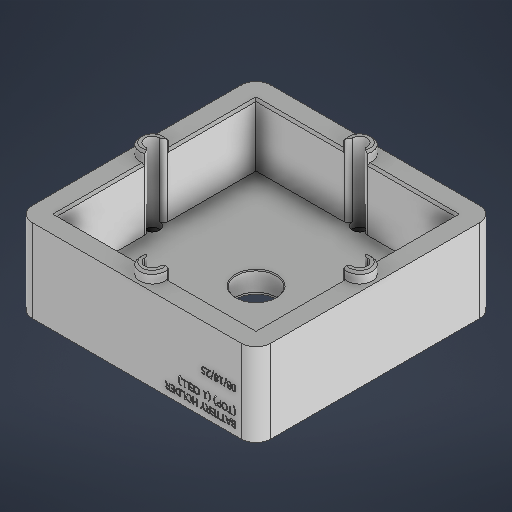
# Autodesk Inventor part: Battery Holder (Top)
Saved by Autodesk Inventor 2025 (Build 290162000, 162)
## iProperties
Created: 2025-08-08
Part Number: Battery Holder (Top)
Material: Generic
Document SubType Name: Modeling
Designer: mayhe
Density: 1 g/cm^3
Appearance: Default
Author: mayhe
Autodesk Inventor part; units mm, degrees
ref_plane "YZ Plane" through (0, 0, 0) normal (1, 0, 0) x (0, 1, 0)
ref_plane "XZ Plane" through (0, 0, 0) normal (0, 1, 0) x (-1, 0, 0)
ref_plane "XY Plane" through (0, 0, 0) normal (0, 0, 1) x (1, 0, 0)
sketch "Sketch1" plane through (0, 0, 0) normal (0, 1, 0) x (-1, 0, 0)
  line L0 (57.5, 57.5) -> (-57.5, 57.5)
  line L1 (-57.5, 57.5) -> (-57.5, -57.5)
  line L2 (-57.5, -57.5) -> (57.5, -57.5)
  line L3 (57.5, -57.5) -> (57.5, 57.5)
  line L4 (57.5, 57.5) -> (-57.5, -57.5) construction
  line L5 (-57.5, 57.5) -> (57.5, -57.5) construction
  point P0 (0, 0)
  dimension "d0" = 115
  dimension "d1" = 115
  constraints: 12 end point, 2 midpoint, 2 parallel, 1 horizontal, 1 perpendicular
  measures "d0" distance of L2.end L1.end
  measures "d1" distance of L1.end L0.end
extrude "Extrusion1" add sketch "Sketch1" along normal blind 10
sketch "Sketch4" plane through (0, 10, 0) normal (0, 1, 0) x (1, 0, 0)
  line L0 (-48, -48) -> (48, -48)
  line L1 (48, -48) -> (48, 48)
  line L2 (48, 48) -> (-48, 48)
  line L3 (-48, 48) -> (-48, -48)
  line L4 (-57.5, 57.5) -> (-57.5, -57.5) projected
  line L5 (-57.5, 0) -> (-48, 0)
  line L6 (-57.5, -57.5) -> (57.5, -57.5) projected
  line L7 (-57.5, 57.5) -> (57.5, 57.5)
  line L8 (57.5, 57.5) -> (57.5, -57.5)
  line L9 (57.5, -57.5) -> (-57.5, -57.5)
  line L10 (-57.5, -57.5) -> (-57.5, 57.5)
  circle A0 centre (0, 0) radius 9.5
  point P0 (47.3285, -94.6135)
  point P1 (-53.5957, 219.1108)
  point P2 (48, 0)
  point P3 (0, -48)
  point P4 (0, -57.5)
  dimension "d48" = 96
  dimension "d49" = 96
  dimension "d217" = 19
  constraints: 18 end point, 6 midpoint, 4 parallel, 2 horizontal, 2 perpendicular, 1 centre point, 1 horizontal alignment, 1 vertical alignment
  measures "d48" distance of L2.end L1.end
  measures "d49" distance of L1.end L0.end
  measures "d217" diameter of A0
extrude "Extrusion3" add sketch "Sketch4" along normal blind 30 contours L7 L8 L6 L4
hole "Hole4" at (0, 10, 0) direction (0, -1, 0) diameter 18.6 end through all countersink diameter 19 countersink angle 2.5
sketch "Sketch6" plane through (0, 0, 0) normal (0, -1, 0) x (1, 0, 0)
  line L0 (50, 50) -> (-50, 50)
  line L1 (-50, 50) -> (-50, -50)
  line L2 (-50, -50) -> (50, -50)
  line L3 (50, -50) -> (50, 50)
  line L4 (50, 50) -> (-50, -50) construction
  line L5 (-50, 50) -> (50, -50) construction
  circle A0 centre (-50, -50) radius 3
  circle A1 centre (0, -50) radius 3
  circle A2 centre (50, -50) radius 3
  circle A3 centre (-50, 0) radius 3
  circle A4 centre (0, 0) radius 3
  circle A5 centre (50, 0) radius 3
  circle A6 centre (-50, 50) radius 3
  circle A7 centre (0, 50) radius 3
  circle A8 centre (50, 50) radius 3
  dimension "d183" = 100
  dimension "d184" = 100
  dimension "d185" = 6
  dimension "d188" = 50
  dimension "d191" = 50
  constraints: 12 end point, 9 centre point, 2 horizontal, 2 midpoint, 2 parallel, 1 coincident, 1 perpendicular, 1 vertical, 16 other
  measures "d183" distance of L2.end L1.end
  measures "d184" distance of L1.end L0.end
  measures "d185" diameter of A0
  measures "d188" distance of A0.centre A1.centre
  measures "d191" distance of A0.centre A3.centre
hole "Hole5" at (-50, 0, 0) at (0, 0, -50) at (50, 0, 0) at (0, 0, 50) direction (0, 1, 0) diameter 7.125 end through all counterbore diameter 13 counterbore depth 7
sketch "Sketch7" plane through (0, 40, 0) normal (0, 1, 0) x (1, 0, 0)
  arc A0 (-48, 2.9481) -> (-48, -2.9481) centre (-50, 0) ccw projected
  arc A1 (-48, 5.6569) -> (-48, -5.6569) centre (-50, 0) ccw
  circle A2 centre (50, 0) radius 6.5 projected
  arc A3 (48, -5.6569) -> (48, 5.6569) centre (50, 0) ccw
  circle A4 centre (0, 50) radius 3.5625 projected
  arc A5 (5.6569, 48) -> (-5.6569, 48) centre (0, 50) ccw
  arc A6 (-2.9481, -48) -> (2.9481, -48) centre (0, -50) ccw projected
  arc A7 (-5.6569, -48) -> (5.6569, -48) centre (0, -50) ccw
  line L0 (-2.9481, 48) -> (-48, 48) projected
  line L1 (48, -48) -> (2.9481, -48) projected
  line L2 (-48, 48) -> (48, 48)
  line L3 (48, 48) -> (48, -48)
  line L4 (48, -48) -> (-48, -48)
  line L5 (-48, -48) -> (-48, 48)
  arc A8 (-48, 2.9481) -> (-48, -2.9481) centre (-50, 0) ccw
  arc A9 (-2.9481, -48) -> (2.9481, -48) centre (0, -50) ccw
  arc A10 (48, -2.9481) -> (48, 2.9481) centre (50, 0) ccw
  arc A11 (2.9481, 48) -> (-2.9481, 48) centre (0, 50) ccw
  point P0 (0, 0)
  point P1 (-48, 2.9481)
  point P2 (-48, -2.9481)
  point P3 (-2.9481, -48)
  point P4 (5.6569, -48)
  point P5 (-5.6569, 48)
  dimension "d201" = 12
  dimension "d202" = 12
  dimension "d203" = 12
  dimension "d204" = 12
  constraints: 16 point on circle, 16 point on line, 8 centre point, 8 coincident, 8 end point, 2 concentric, 2 parallel, 1 horizontal, 1 perpendicular, 2 other
  measures "d201" diameter of A1
  measures "d202" diameter of A3
  measures "d203" diameter of A5
  measures "d204" diameter of A7
extrude "Extrusion4" add sketch "Sketch7" along normal blind 5 contours A0 L5 A1 | A5 L2 A4 L0 | L4 A6 L1 A7 | A3 L3 A10
fillet "Fillet1" radius 7.125 4 edges at (-57.5, 20, -57.5) (57.5, 20, -57.5) (57.5, 20, 57.5) (-57.5, 20, 57.5)
fillet "Fillet2" radius 2 16 edges at (2.9481, 25, -48) (-2.9481, 42.5, -48) (-2.9481, 25, -48) (2.9481, 42.5, -48) (48, 25, 2.9481) (48, 42.5, -2.9481) (48, 25, -2.9481) (48, 42.5, 2.9481) (2.9481, 42.5, 48) (2.9481, 25, 48) (-2.9481, 25, 48) (-2.9481, 42.5, 48) (-48, 25, -2.9481) (-48, 42.5, 2.9481) (-48, 25, 2.9481) (-48, 42.5, -2.9481)
chamfer "Chamfer1" distance 0.4 angle 45 1 edges at (0, 10, -9.5)
chamfer "Chamfer2" distance 1 angle 45 12 edges at (0, 45, -56) (-56, 45, 0) (0, 45, 56) (56, 45, 0) (-26.8284, 40, -48) (-48, 40, -26.8284) (48, 40, -26.8284) (26.8284, 40, -48) (48, 40, 26.8284) (26.8284, 40, 48) (-26.8284, 40, 48) (-48, 40, 26.8284)
sketch "Sketch8" plane through (-50.375, 0, 57.5) normal (0, 0, 1) x (1, 0, 0)
  line L0 (98.2962, 2.8919) -> (49.8661, 2.8919) construction
  line L1 (49.8661, 2.8919) -> (49.8661, 31.9849) construction
  line L2 (49.8661, 31.9849) -> (98.2962, 31.9849) construction
  line L3 (98.2962, 31.9849) -> (98.2962, 2.8919) construction
  spline S0 degree 2 poles (95.92, 5.068) (95.92, 5.2953) (96.0929, 5.6435) (96.2362, 5.7572) knots 0 0 0 1 2 2 2
  spline S1 degree 2 poles (96.2362, 5.7572) (96.4091, 5.8905) (96.8018, 6.0042) (97.113, 6.0042) knots 0 0 0 1 2 2 2
  line L4 (97.113, 6.0042) -> (97.9874, 6.0042)
  line L5 (97.9874, 6.0042) -> (97.9874, 2.9562)
  line L6 (97.9874, 2.9562) -> (97.1797, 2.9562)
  spline S2 degree 2 poles (97.1797, 2.9562) (96.8537, 2.9562) (96.5276, 2.9981) (96.3794, 3.0797) knots 0 0 0 1 2 2 2
  spline S3 degree 2 poles (96.3794, 3.0797) (96.2139, 3.1661) (96.0633, 3.4502) (96.0633, 3.6428) knots 0 0 0 1 2 2 2
  spline S4 degree 2 poles (96.0633, 3.6428) (96.0633, 3.8577) (96.2905, 4.1986) (96.4906, 4.2949) knots 0 0 0 1 2 2 2
  line L7 (96.4906, 4.2949) -> (96.4906, 4.3097)
  spline S5 degree 2 poles (96.4906, 4.3097) (96.2189, 4.3838) (95.92, 4.7766) (95.92, 5.068) knots 0 0 0 1 2 2 2
  spline S6 degree 2 poles (96.3424, 5.0853) (96.3424, 4.9124) (96.4412, 4.6901) (96.5894, 4.6111) knots 0 0 0 1 2 2 2
  spline S7 degree 2 poles (96.5894, 4.6111) (96.6857, 4.5617) (96.913, 4.532) (97.1229, 4.532) knots 0 0 0 1 2 2 2
  line L8 (97.1229, 4.532) -> (97.5823, 4.532)
  line L9 (97.5823, 4.532) -> (97.5823, 5.6584)
  line L10 (97.5823, 5.6584) -> (97.2538, 5.6584)
  spline S8 degree 2 poles (97.2538, 5.6584) (96.9871, 5.6584) (96.6808, 5.609) (96.5622, 5.5299) knots 0 0 0 1 2 2 2
  spline S9 degree 2 poles (96.5622, 5.5299) (96.4486, 5.4484) (96.3424, 5.2459) (96.3424, 5.0853) knots 0 0 0 1 2 2 2
  spline S10 degree 2 poles (96.4856, 3.6996) (96.4856, 3.591) (96.5598, 3.4279) (96.6413, 3.381) knots 0 0 0 1 2 2 2
  spline S11 degree 2 poles (96.6413, 3.381) (96.7401, 3.3267) (96.9797, 3.302) (97.1945, 3.302) knots 0 0 0 1 2 2 2
  line L11 (97.1945, 3.302) -> (97.5823, 3.302)
  line L12 (97.5823, 3.302) -> (97.5823, 4.1936)
  line L13 (97.5823, 4.1936) -> (97.1229, 4.1936)
  spline S12 degree 2 poles (97.1229, 4.1936) (96.9327, 4.1936) (96.7524, 4.1541) (96.6561, 4.0924) knots 0 0 0 1 2 2 2
  spline S13 degree 2 poles (96.6561, 4.0924) (96.5622, 4.0331) (96.4856, 3.8429) (96.4856, 3.6996) knots 0 0 0 1 2 2 2
  line L14 (95.8459, 6.0042) -> (94.8184, 2.9562)
  line L15 (94.8184, 2.9562) -> (94.3194, 2.9562)
  line L16 (94.3194, 2.9562) -> (93.2919, 6.0042)
  line L17 (93.2919, 6.0042) -> (93.7192, 6.0042)
  line L18 (93.7192, 6.0042) -> (93.9959, 5.152)
  line L19 (93.9959, 5.152) -> (95.1593, 5.152)
  line L20 (95.1593, 5.152) -> (95.4359, 6.0042)
  line L21 (95.4359, 6.0042) -> (95.8459, 6.0042)
  line L22 (94.107, 4.8062) -> (94.5788, 3.3711)
  line L23 (94.5788, 3.3711) -> (95.0481, 4.8062)
  line L24 (95.0481, 4.8062) -> (94.107, 4.8062)
  line L25 (92.2916, 6.0042) -> (92.2916, 3.3168)
  line L26 (92.2916, 3.3168) -> (93.3141, 3.3168)
  line L27 (93.3141, 3.3168) -> (93.3141, 2.9562)
  line L28 (93.3141, 2.9562) -> (90.8639, 2.9562)
  line L29 (90.8639, 2.9562) -> (90.8639, 3.3168)
  line L30 (90.8639, 3.3168) -> (91.8865, 3.3168)
  line L31 (91.8865, 3.3168) -> (91.8865, 6.0042)
  line L32 (91.8865, 6.0042) -> (92.2916, 6.0042)
  line L33 (89.8438, 6.0042) -> (89.8438, 3.3168)
  line L34 (89.8438, 3.3168) -> (90.8664, 3.3168)
  line L35 (90.8664, 3.3168) -> (90.8664, 2.9562)
  line L36 (90.8664, 2.9562) -> (88.4161, 2.9562)
  line L37 (88.4161, 2.9562) -> (88.4161, 3.3168)
  line L38 (88.4161, 3.3168) -> (89.4387, 3.3168)
  line L39 (89.4387, 3.3168) -> (89.4387, 6.0042)
  line L40 (89.4387, 6.0042) -> (89.8438, 6.0042)
  line L41 (88.1074, 6.0042) -> (88.1074, 2.9562)
  line L42 (88.1074, 2.9562) -> (86.2005, 2.9562)
  line L43 (86.2005, 2.9562) -> (86.2005, 3.3168)
  line L44 (86.2005, 3.3168) -> (87.7023, 3.3168)
  line L45 (87.7023, 3.3168) -> (87.7023, 4.1516)
  line L46 (87.7023, 4.1516) -> (86.3018, 4.1516)
  line L47 (86.3018, 4.1516) -> (86.3018, 4.5123)
  line L48 (86.3018, 4.5123) -> (87.7023, 4.5123)
  line L49 (87.7023, 4.5123) -> (87.7023, 5.6435)
  line L50 (87.7023, 5.6435) -> (86.2005, 5.6435)
  line L51 (86.2005, 5.6435) -> (86.2005, 6.0042)
  line L52 (86.2005, 6.0042) -> (88.1074, 6.0042)
  line L53 (83.397, 6.0042) -> (83.9231, 6.0042)
  line L54 (83.9231, 6.0042) -> (84.8865, 4.7914)
  line L55 (84.8865, 4.7914) -> (85.3508, 4.7914)
  line L56 (85.3508, 4.7914) -> (85.3508, 6.0042)
  line L57 (85.3508, 6.0042) -> (85.7559, 6.0042)
  line L58 (85.7559, 6.0042) -> (85.7559, 2.9562)
  line L59 (85.7559, 2.9562) -> (84.9704, 2.9562)
  spline S14 degree 2 poles (84.9704, 2.9562) (84.7086, 2.9562) (84.3554, 3.013) (84.1948, 3.1167) knots 0 0 0 1 2 2 2
  spline S15 degree 2 poles (84.1948, 3.1167) (84.0343, 3.2204) (83.849, 3.544) (83.849, 3.7836) knots 0 0 0 1 2 2 2
  spline S16 degree 2 poles (83.849, 3.7836) (83.849, 4.1171) (84.1899, 4.5691) (84.4814, 4.6778) knots 0 0 0 1 2 2 2
  line L60 (84.4814, 4.6778) -> (83.397, 6.0042)
  spline S17 degree 2 poles (84.2714, 3.8157) (84.2714, 3.6823) (84.3653, 3.4773) (84.4641, 3.4106) knots 0 0 0 1 2 2 2
  spline S18 degree 2 poles (84.4641, 3.4106) (84.5505, 3.3538) (84.7802, 3.3069) (84.9482, 3.3069) knots 0 0 0 1 2 2 2
  line L61 (84.9482, 3.3069) -> (85.3508, 3.3069)
  line L62 (85.3508, 3.3069) -> (85.3508, 4.453)
  line L63 (85.3508, 4.453) -> (84.9951, 4.453)
  spline S19 degree 2 poles (84.9951, 4.453) (84.8198, 4.453) (84.5407, 4.3912) (84.4443, 4.2949) knots 0 0 0 1 2 2 2
  spline S20 degree 2 poles (84.4443, 4.2949) (84.3554, 4.2109) (84.2714, 3.9738) (84.2714, 3.8157) knots 0 0 0 1 2 2 2
  line L64 (81.0209, 2.9562) -> (82.0509, 4.6555)
  line L65 (82.0509, 4.6555) -> (82.0509, 6.0042)
  line L66 (82.0509, 6.0042) -> (82.456, 6.0042)
  line L67 (82.456, 6.0042) -> (82.456, 4.6975)
  line L68 (82.456, 4.6975) -> (83.486, 2.9562)
  line L69 (83.486, 2.9562) -> (83.0364, 2.9562)
  line L70 (83.0364, 2.9562) -> (82.2485, 4.2974)
  line L71 (82.2485, 4.2974) -> (81.4507, 2.9562)
  line L72 (81.4507, 2.9562) -> (81.0209, 2.9562)
  line L73 (77.2171, 6.0042) -> (77.6221, 6.0042)
  line L74 (77.6221, 6.0042) -> (77.6221, 4.5123)
  line L75 (77.6221, 4.5123) -> (79.0251, 4.5123)
  line L76 (79.0251, 4.5123) -> (79.0251, 6.0042)
  line L77 (79.0251, 6.0042) -> (79.4302, 6.0042)
  line L78 (79.4302, 6.0042) -> (79.4302, 2.9562)
  line L79 (79.4302, 2.9562) -> (79.0251, 2.9562)
  line L80 (79.0251, 2.9562) -> (79.0251, 4.1516)
  line L81 (79.0251, 4.1516) -> (77.6221, 4.1516)
  line L82 (77.6221, 4.1516) -> (77.6221, 2.9562)
  line L83 (77.6221, 2.9562) -> (77.2171, 2.9562)
  line L84 (77.2171, 2.9562) -> (77.2171, 6.0042)
  spline S21 degree 2 poles (74.4432, 3.3044) (74.2703, 3.507) (74.0777, 4.0998) (74.0777, 4.4802) knots 0 0 0 1 2 2 2
  spline S22 degree 2 poles (74.0777, 4.4802) (74.0777, 4.8507) (74.2654, 5.4509) (74.4432, 5.6534) knots 0 0 0 1 2 2 2
  spline S23 degree 2 poles (74.4432, 5.6534) (74.6309, 5.8658) (75.1274, 6.0684) (75.4263, 6.0684) knots 0 0 0 1 2 2 2
  spline S24 degree 2 poles (75.4263, 6.0684) (75.735, 6.0684) (76.229, 5.8584) (76.4094, 5.6534) knots 0 0 0 1 2 2 2
  spline S25 degree 2 poles (76.4094, 5.6534) (76.5847, 5.4509) (76.7725, 4.8556) (76.7725, 4.4802) knots 0 0 0 1 2 2 2
  spline S26 degree 2 poles (76.7725, 4.4802) (76.7725, 4.0973) (76.5823, 3.5144) (76.4069, 3.3044) knots 0 0 0 1 2 2 2
  spline S27 degree 2 poles (76.4069, 3.3044) (76.229, 3.1019) (75.7326, 2.8919) (75.4263, 2.8919) knots 0 0 0 1 2 2 2
  spline S28 degree 2 poles (75.4263, 2.8919) (75.1151, 2.8919) (74.6161, 3.1093) (74.4432, 3.3044) knots 0 0 0 1 2 2 2
  spline S29 degree 2 poles (74.5, 4.4802) (74.5, 4.1788) (74.6309, 3.712) (74.7495, 3.5588) knots 0 0 0 1 2 2 2
  spline S30 degree 2 poles (74.7495, 3.5588) (74.8705, 3.4008) (75.2114, 3.2427) (75.4238, 3.2427) knots 0 0 0 1 2 2 2
  spline S31 degree 2 poles (75.4238, 3.2427) (75.6437, 3.2427) (75.9746, 3.3958) (76.1006, 3.5588) knots 0 0 0 1 2 2 2
  spline S32 degree 2 poles (76.1006, 3.5588) (76.2216, 3.7145) (76.3501, 4.1838) (76.3501, 4.4802) knots 0 0 0 1 2 2 2
  spline S33 degree 2 poles (76.3501, 4.4802) (76.3501, 5.0804) (75.8462, 5.7176) (75.4238, 5.7176) knots 0 0 0 1 2 2 2
  spline S34 degree 2 poles (75.4238, 5.7176) (75.0014, 5.7176) (74.5, 5.0804) (74.5, 4.4802) knots 0 0 0 1 2 2 2
  line L85 (71.867, 6.0042) -> (73.6331, 6.0042)
  line L86 (73.6331, 6.0042) -> (73.6331, 2.9562)
  line L87 (73.6331, 2.9562) -> (73.228, 2.9562)
  line L88 (73.228, 2.9562) -> (73.228, 5.6435)
  line L89 (73.228, 5.6435) -> (71.867, 5.6435)
  line L90 (71.867, 5.6435) -> (71.867, 6.0042)
  spline S35 degree 2 poles (69.145, 4.4826) (69.145, 4.9001) (69.4834, 5.5719) (69.7675, 5.7596) knots 0 0 0 1 2 2 2
  spline S36 degree 2 poles (69.7675, 5.7596) (69.9997, 5.9054) (70.4764, 6.0042) (70.8469, 6.0042) knots 0 0 0 1 2 2 2
  line L91 (70.8469, 6.0042) -> (71.5484, 6.0042)
  line L92 (71.5484, 6.0042) -> (71.5484, 2.9562)
  line L93 (71.5484, 2.9562) -> (70.8543, 2.9562)
  spline S37 degree 2 poles (70.8543, 2.9562) (70.4245, 2.9562) (69.9354, 3.0846) (69.7625, 3.1982) knots 0 0 0 1 2 2 2
  spline S38 degree 2 poles (69.7625, 3.1982) (69.4686, 3.3933) (69.145, 4.038) (69.145, 4.4826) knots 0 0 0 1 2 2 2
  spline S39 degree 2 poles (69.5674, 4.4777) (69.5674, 4.1269) (69.7996, 3.6305) (70.0293, 3.4897) knots 0 0 0 1 2 2 2
  spline S40 degree 2 poles (70.0293, 3.4897) (70.1923, 3.3933) (70.5604, 3.3069) (70.8345, 3.3069) knots 0 0 0 1 2 2 2
  line L94 (70.8345, 3.3069) -> (71.1433, 3.3069)
  line L95 (71.1433, 3.3069) -> (71.1433, 5.6534)
  line L96 (71.1433, 5.6534) -> (70.8345, 5.6534)
  spline S41 degree 2 poles (70.8345, 5.6534) (70.5653, 5.6534) (70.1577, 5.567) (69.9923, 5.4509) knots 0 0 0 1 2 2 2
  spline S42 degree 2 poles (69.9923, 5.4509) (69.7798, 5.3076) (69.5674, 4.8334) (69.5674, 4.4777) knots 0 0 0 1 2 2 2
  line L97 (68.7054, 6.0042) -> (68.7054, 2.9562)
  line L98 (68.7054, 2.9562) -> (66.7985, 2.9562)
  line L99 (66.7985, 2.9562) -> (66.7985, 3.3168)
  line L100 (66.7985, 3.3168) -> (68.3003, 3.3168)
  line L101 (68.3003, 3.3168) -> (68.3003, 4.1516)
  line L102 (68.3003, 4.1516) -> (66.8998, 4.1516)
  line L103 (66.8998, 4.1516) -> (66.8998, 4.5123)
  line L104 (66.8998, 4.5123) -> (68.3003, 4.5123)
  line L105 (68.3003, 4.5123) -> (68.3003, 5.6435)
  line L106 (68.3003, 5.6435) -> (66.7985, 5.6435)
  line L107 (66.7985, 5.6435) -> (66.7985, 6.0042)
  line L108 (66.7985, 6.0042) -> (68.7054, 6.0042)
  line L109 (63.9951, 6.0042) -> (64.5212, 6.0042)
  line L110 (64.5212, 6.0042) -> (65.4845, 4.7914)
  line L111 (65.4845, 4.7914) -> (65.9488, 4.7914)
  line L112 (65.9488, 4.7914) -> (65.9488, 6.0042)
  line L113 (65.9488, 6.0042) -> (66.3539, 6.0042)
  line L114 (66.3539, 6.0042) -> (66.3539, 2.9562)
  line L115 (66.3539, 2.9562) -> (65.5685, 2.9562)
  spline S43 degree 2 poles (65.5685, 2.9562) (65.3066, 2.9562) (64.9534, 3.013) (64.7929, 3.1167) knots 0 0 0 1 2 2 2
  spline S44 degree 2 poles (64.7929, 3.1167) (64.6323, 3.2204) (64.4471, 3.544) (64.4471, 3.7836) knots 0 0 0 1 2 2 2
  spline S45 degree 2 poles (64.4471, 3.7836) (64.4471, 4.1171) (64.7879, 4.5691) (65.0794, 4.6778) knots 0 0 0 1 2 2 2
  line L116 (65.0794, 4.6778) -> (63.9951, 6.0042)
  spline S46 degree 2 poles (64.8694, 3.8157) (64.8694, 3.6823) (64.9633, 3.4773) (65.0621, 3.4106) knots 0 0 0 1 2 2 2
  spline S47 degree 2 poles (65.0621, 3.4106) (65.1486, 3.3538) (65.3783, 3.3069) (65.5462, 3.3069) knots 0 0 0 1 2 2 2
  line L117 (65.5462, 3.3069) -> (65.9488, 3.3069)
  line L118 (65.9488, 3.3069) -> (65.9488, 4.453)
  line L119 (65.9488, 4.453) -> (65.5932, 4.453)
  spline S48 degree 2 poles (65.5932, 4.453) (65.4178, 4.453) (65.1387, 4.3912) (65.0423, 4.2949) knots 0 0 0 1 2 2 2
  spline S49 degree 2 poles (65.0423, 4.2949) (64.9534, 4.2109) (64.8694, 3.9738) (64.8694, 3.8157) knots 0 0 0 1 2 2 2
  line L120 (96.8438, 11.8649) -> (97.3131, 11.8649)
  spline S50 degree 2 poles (97.3131, 11.8649) (97.6688, 11.4425) (98.0763, 10.4965) (98.0763, 9.8518) knots 0 0 0 1 2 2 2
  spline S51 degree 2 poles (98.0763, 9.8518) (98.0763, 9.222) (97.6737, 8.2611) (97.3131, 7.8388) knots 0 0 0 1 2 2 2
  line L121 (97.3131, 7.8388) -> (96.8438, 7.8388)
  line L122 (96.8438, 7.8388) -> (96.8438, 7.8585)
  spline S52 degree 2 poles (96.8438, 7.8585) (97.0093, 8.0092) (97.3106, 8.3995) (97.4391, 8.6588) knots 0 0 0 1 2 2 2
  spline S53 degree 2 poles (97.4391, 8.6588) (97.5626, 8.9107) (97.7157, 9.5159) (97.7157, 9.8518) knots 0 0 0 1 2 2 2
  spline S54 degree 2 poles (97.7157, 9.8518) (97.7157, 10.2026) (97.5675, 10.783) (97.4391, 11.0448) knots 0 0 0 1 2 2 2
  spline S55 degree 2 poles (97.4391, 11.0448) (97.3156, 11.2968) (97.0019, 11.7043) (96.8438, 11.8451) knots 0 0 0 1 2 2 2
  line L123 (96.8438, 11.8451) -> (96.8438, 11.8649)
  line L124 (95.6705, 11.0226) -> (95.6705, 8.3352)
  line L125 (95.6705, 8.3352) -> (96.6931, 8.3352)
  line L126 (96.6931, 8.3352) -> (96.6931, 7.9746)
  line L127 (96.6931, 7.9746) -> (94.2429, 7.9746)
  line L128 (94.2429, 7.9746) -> (94.2429, 8.3352)
  line L129 (94.2429, 8.3352) -> (95.2655, 8.3352)
  line L130 (95.2655, 8.3352) -> (95.2655, 11.0226)
  line L131 (95.2655, 11.0226) -> (95.6705, 11.0226)
  spline S56 degree 2 poles (91.7778, 8.3229) (91.6049, 8.5254) (91.4122, 9.1182) (91.4122, 9.4986) knots 0 0 0 1 2 2 2
  spline S57 degree 2 poles (91.4122, 9.4986) (91.4122, 9.8691) (91.6, 10.4693) (91.7778, 10.6719) knots 0 0 0 1 2 2 2
  spline S58 degree 2 poles (91.7778, 10.6719) (91.9655, 10.8843) (92.462, 11.0868) (92.7609, 11.0868) knots 0 0 0 1 2 2 2
  spline S59 degree 2 poles (92.7609, 11.0868) (93.0696, 11.0868) (93.5636, 10.8769) (93.7439, 10.6719) knots 0 0 0 1 2 2 2
  spline S60 degree 2 poles (93.7439, 10.6719) (93.9193, 10.4693) (94.107, 9.8741) (94.107, 9.4986) knots 0 0 0 1 2 2 2
  spline S61 degree 2 poles (94.107, 9.4986) (94.107, 9.1158) (93.9168, 8.5328) (93.7415, 8.3229) knots 0 0 0 1 2 2 2
  spline S62 degree 2 poles (93.7415, 8.3229) (93.5636, 8.1203) (93.0671, 7.9104) (92.7609, 7.9104) knots 0 0 0 1 2 2 2
  spline S63 degree 2 poles (92.7609, 7.9104) (92.4496, 7.9104) (91.9507, 8.1277) (91.7778, 8.3229) knots 0 0 0 1 2 2 2
  spline S64 degree 2 poles (91.8346, 9.4986) (91.8346, 9.1973) (91.9655, 8.7304) (92.0841, 8.5773) knots 0 0 0 1 2 2 2
  spline S65 degree 2 poles (92.0841, 8.5773) (92.2051, 8.4192) (92.546, 8.2611) (92.7584, 8.2611) knots 0 0 0 1 2 2 2
  spline S66 degree 2 poles (92.7584, 8.2611) (92.9782, 8.2611) (93.3092, 8.4143) (93.4352, 8.5773) knots 0 0 0 1 2 2 2
  spline S67 degree 2 poles (93.4352, 8.5773) (93.5562, 8.7329) (93.6847, 9.2022) (93.6847, 9.4986) knots 0 0 0 1 2 2 2
  spline S68 degree 2 poles (93.6847, 9.4986) (93.6847, 10.0988) (93.1808, 10.7361) (92.7584, 10.7361) knots 0 0 0 1 2 2 2
  spline S69 degree 2 poles (92.7584, 10.7361) (92.336, 10.7361) (91.8346, 10.0988) (91.8346, 9.4986) knots 0 0 0 1 2 2 2
  spline S70 degree 2 poles (89.041, 8.8935) (89.041, 9.0911) (89.1818, 9.4467) (89.3078, 9.5702) knots 0 0 0 1 2 2 2
  spline S71 degree 2 poles (89.3078, 9.5702) (89.4659, 9.7258) (89.8932, 9.8864) (90.2192, 9.8864) knots 0 0 0 1 2 2 2
  line L132 (90.2192, 9.8864) -> (90.5626, 9.8864)
  line L133 (90.5626, 9.8864) -> (90.5626, 11.0226)
  line L134 (90.5626, 11.0226) -> (90.9676, 11.0226)
  line L135 (90.9676, 11.0226) -> (90.9676, 7.9746)
  line L136 (90.9676, 7.9746) -> (90.2019, 7.9746)
  spline S72 degree 2 poles (90.2019, 7.9746) (89.9302, 7.9746) (89.5498, 8.0635) (89.4041, 8.1648) knots 0 0 0 1 2 2 2
  spline S73 degree 2 poles (89.4041, 8.1648) (89.2337, 8.2809) (89.041, 8.639) (89.041, 8.8935) knots 0 0 0 1 2 2 2
  spline S74 degree 2 poles (89.4634, 8.9058) (89.4634, 8.7477) (89.5721, 8.5155) (89.6832, 8.4414) knots 0 0 0 1 2 2 2
  spline S75 degree 2 poles (89.6832, 8.4414) (89.7796, 8.3772) (90.0364, 8.3254) (90.2266, 8.3254) knots 0 0 0 1 2 2 2
  line L137 (90.2266, 8.3254) -> (90.5626, 8.3254)
  line L138 (90.5626, 8.3254) -> (90.5626, 9.5406)
  line L139 (90.5626, 9.5406) -> (90.2859, 9.5406)
  spline S76 degree 2 poles (90.2859, 9.5406) (90.0389, 9.5406) (89.7351, 9.4616) (89.6363, 9.3578) knots 0 0 0 1 2 2 2
  spline S77 degree 2 poles (89.6363, 9.3578) (89.5449, 9.2664) (89.4634, 9.0515) (89.4634, 8.9058) knots 0 0 0 1 2 2 2
  spline S78 degree 2 poles (87.5788, 9.8518) (87.5788, 10.4841) (87.9839, 11.4425) (88.342, 11.8649) knots 0 0 0 1 2 2 2
  line L140 (88.342, 11.8649) -> (88.8113, 11.8649)
  line L141 (88.8113, 11.8649) -> (88.8113, 11.8451)
  spline S79 degree 2 poles (88.8113, 11.8451) (88.6532, 11.7043) (88.3346, 11.2918) (88.216, 11.0448) knots 0 0 0 1 2 2 2
  spline S80 degree 2 poles (88.216, 11.0448) (88.0876, 10.7805) (87.9394, 10.1927) (87.9394, 9.8518) knots 0 0 0 1 2 2 2
  spline S81 degree 2 poles (87.9394, 9.8518) (87.9394, 9.5134) (88.0901, 8.9132) (88.216, 8.6588) knots 0 0 0 1 2 2 2
  spline S82 degree 2 poles (88.216, 8.6588) (88.3395, 8.4044) (88.6557, 7.9993) (88.8113, 7.8585) knots 0 0 0 1 2 2 2
  line L142 (88.8113, 7.8585) -> (88.8113, 7.8388)
  line L143 (88.8113, 7.8388) -> (88.342, 7.8388)
  spline S83 degree 2 poles (88.342, 7.8388) (87.9863, 8.2611) (87.5788, 9.2146) (87.5788, 9.8518) knots 0 0 0 1 2 2 2
  line L144 (84.5975, 11.8649) -> (85.0668, 11.8649)
  spline S84 degree 2 poles (85.0668, 11.8649) (85.4224, 11.4425) (85.83, 10.4965) (85.83, 9.8518) knots 0 0 0 1 2 2 2
  spline S85 degree 2 poles (85.83, 9.8518) (85.83, 9.222) (85.4274, 8.2611) (85.0668, 7.8388) knots 0 0 0 1 2 2 2
  line L145 (85.0668, 7.8388) -> (84.5975, 7.8388)
  line L146 (84.5975, 7.8388) -> (84.5975, 7.8585)
  spline S86 degree 2 poles (84.5975, 7.8585) (84.763, 8.0092) (85.0643, 8.3995) (85.1927, 8.6588) knots 0 0 0 1 2 2 2
  spline S87 degree 2 poles (85.1927, 8.6588) (85.3162, 8.9107) (85.4694, 9.5159) (85.4694, 9.8518) knots 0 0 0 1 2 2 2
  spline S88 degree 2 poles (85.4694, 9.8518) (85.4694, 10.2026) (85.3212, 10.783) (85.1927, 11.0448) knots 0 0 0 1 2 2 2
  spline S89 degree 2 poles (85.1927, 11.0448) (85.0692, 11.2968) (84.7555, 11.7043) (84.5975, 11.8451) knots 0 0 0 1 2 2 2
  line L147 (84.5975, 11.8451) -> (84.5975, 11.8649)
  line L148 (82.4955, 11.0226) -> (83.9824, 11.0226)
  line L149 (83.9824, 11.0226) -> (83.9824, 10.7114)
  line L150 (83.9824, 10.7114) -> (83.4291, 10.7114)
  line L151 (83.4291, 10.7114) -> (83.4291, 8.6687)
  line L152 (83.4291, 8.6687) -> (83.9824, 8.6687)
  line L153 (83.9824, 8.6687) -> (83.9824, 8.3896)
  spline S90 degree 2 poles (83.9824, 8.3896) (83.6687, 8.3896) (83.3723, 8.2117) (83.3526, 7.9647) knots 0 0 0 1 2 2 2
  line L154 (83.3526, 7.9647) -> (83.0364, 7.9647)
  line L155 (83.0364, 7.9647) -> (83.0364, 10.7114)
  line L156 (83.0364, 10.7114) -> (82.4955, 10.7114)
  line L157 (82.4955, 10.7114) -> (82.4955, 11.0226)
  spline S91 degree 2 poles (79.3487, 11.0769) (79.6451, 11.0769) (80.1465, 10.8769) (80.3293, 10.6768) knots 0 0 0 1 2 2 2
  spline S92 degree 2 poles (80.3293, 10.6768) (80.5121, 10.4792) (80.7121, 9.8864) (80.7121, 9.5011) knots 0 0 0 1 2 2 2
  spline S93 degree 2 poles (80.7121, 9.5011) (80.7121, 9.1182) (80.517, 8.5501) (80.3317, 8.3402) knots 0 0 0 1 2 2 2
  spline S94 degree 2 poles (80.3317, 8.3402) (80.149, 8.1352) (79.65, 7.9203) (79.3413, 7.9203) knots 0 0 0 1 2 2 2
  spline S95 degree 2 poles (79.3413, 7.9203) (79.1881, 7.9203) (78.9189, 7.9647) (78.8053, 7.9993) knots 0 0 0 1 2 2 2
  spline S96 degree 2 poles (78.8053, 7.9993) (78.7065, 8.0314) (78.5015, 8.1228) (78.4002, 8.1771) knots 0 0 0 1 2 2 2
  line L158 (78.4002, 8.1771) -> (78.4002, 8.6662)
  line L159 (78.4002, 8.6662) -> (78.4323, 8.6662)
  spline S97 degree 2 poles (78.4323, 8.6662) (78.4866, 8.6168) (78.6546, 8.4785) (78.7756, 8.4118) knots 0 0 0 1 2 2 2
  spline S98 degree 2 poles (78.7756, 8.4118) (78.8917, 8.3476) (79.1659, 8.2661) (79.3437, 8.2661) knots 0 0 0 1 2 2 2
  spline S99 degree 2 poles (79.3437, 8.2661) (79.5389, 8.2661) (79.8871, 8.4266) (80.0181, 8.5798) knots 0 0 0 1 2 2 2
  spline S100 degree 2 poles (80.0181, 8.5798) (80.1465, 8.7354) (80.2898, 9.2071) (80.2898, 9.5011) knots 0 0 0 1 2 2 2
  spline S101 degree 2 poles (80.2898, 9.5011) (80.2898, 9.8148) (80.1391, 10.2668) (80.0082, 10.4224) knots 0 0 0 1 2 2 2
  spline S102 degree 2 poles (80.0082, 10.4224) (79.8797, 10.5731) (79.5364, 10.7262) (79.3437, 10.7262) knots 0 0 0 1 2 2 2
  spline S103 degree 2 poles (79.3437, 10.7262) (79.1684, 10.7262) (78.8695, 10.6398) (78.7534, 10.5755) knots 0 0 0 1 2 2 2
  spline S104 degree 2 poles (78.7534, 10.5755) (78.6423, 10.5113) (78.4768, 10.3779) (78.4298, 10.331) knots 0 0 0 1 2 2 2
  line L160 (78.4298, 10.331) -> (78.4002, 10.331)
  line L161 (78.4002, 10.331) -> (78.4002, 10.8151)
  spline S105 degree 2 poles (78.4002, 10.8151) (78.5015, 10.8621) (78.6793, 10.9485) (78.8053, 10.988) knots 0 0 0 1 2 2 2
  spline S106 degree 2 poles (78.8053, 10.988) (78.9387, 11.0325) (79.1659, 11.0769) (79.3487, 11.0769) knots 0 0 0 1 2 2 2
  line L162 (78.0223, 11.0226) -> (78.0223, 7.9746)
  line L163 (78.0223, 7.9746) -> (76.1154, 7.9746)
  line L164 (76.1154, 7.9746) -> (76.1154, 8.3352)
  line L165 (76.1154, 8.3352) -> (77.6172, 8.3352)
  line L166 (77.6172, 8.3352) -> (77.6172, 9.1701)
  line L167 (77.6172, 9.1701) -> (76.2167, 9.1701)
  line L168 (76.2167, 9.1701) -> (76.2167, 9.5307)
  line L169 (76.2167, 9.5307) -> (77.6172, 9.5307)
  line L170 (77.6172, 9.5307) -> (77.6172, 10.662)
  line L171 (77.6172, 10.662) -> (76.1154, 10.662)
  line L172 (76.1154, 10.662) -> (76.1154, 11.0226)
  line L173 (76.1154, 11.0226) -> (78.0223, 11.0226)
  line L174 (73.9048, 11.0226) -> (75.6708, 11.0226)
  line L175 (75.6708, 11.0226) -> (75.6708, 7.9746)
  line L176 (75.6708, 7.9746) -> (75.2657, 7.9746)
  line L177 (75.2657, 7.9746) -> (75.2657, 10.662)
  line L178 (75.2657, 10.662) -> (73.9048, 10.662)
  line L179 (73.9048, 10.662) -> (73.9048, 11.0226)
  line L180 (71.8201, 11.0226) -> (73.5861, 11.0226)
  line L181 (73.5861, 11.0226) -> (73.5861, 7.9746)
  line L182 (73.5861, 7.9746) -> (73.181, 7.9746)
  line L183 (73.181, 7.9746) -> (73.181, 10.662)
  line L184 (73.181, 10.662) -> (71.8201, 10.662)
  line L185 (71.8201, 10.662) -> (71.8201, 11.0226)
  spline S107 degree 2 poles (70.4245, 9.8518) (70.4245, 10.4841) (70.8296, 11.4425) (71.1877, 11.8649) knots 0 0 0 1 2 2 2
  line L186 (71.1877, 11.8649) -> (71.657, 11.8649)
  line L187 (71.657, 11.8649) -> (71.657, 11.8451)
  spline S108 degree 2 poles (71.657, 11.8451) (71.499, 11.7043) (71.1803, 11.2918) (71.0618, 11.0448) knots 0 0 0 1 2 2 2
  spline S109 degree 2 poles (71.0618, 11.0448) (70.9333, 10.7805) (70.7851, 10.1927) (70.7851, 9.8518) knots 0 0 0 1 2 2 2
  spline S110 degree 2 poles (70.7851, 9.8518) (70.7851, 9.5134) (70.9358, 8.9132) (71.0618, 8.6588) knots 0 0 0 1 2 2 2
  spline S111 degree 2 poles (71.0618, 8.6588) (71.1853, 8.4044) (71.5014, 7.9993) (71.657, 7.8585) knots 0 0 0 1 2 2 2
  line L188 (71.657, 7.8585) -> (71.657, 7.8388)
  line L189 (71.657, 7.8388) -> (71.1877, 7.8388)
  spline S112 degree 2 poles (71.1877, 7.8388) (70.8321, 8.2611) (70.4245, 9.2146) (70.4245, 9.8518) knots 0 0 0 1 2 2 2
  spline S113 degree 2 poles (96.1769, 19.5355) (96.1769, 20.3556) (96.6536, 21.1237) (97.1501, 21.1237) knots 0 0 0 1 2 2 2
  spline S114 degree 2 poles (97.1501, 21.1237) (97.654, 21.1237) (98.1257, 20.3407) (98.1257, 19.538) knots 0 0 0 1 2 2 2
  spline S115 degree 2 poles (98.1257, 19.538) (98.1257, 18.713) (97.649, 17.9498) (97.1501, 17.9498) knots 0 0 0 1 2 2 2
  spline S116 degree 2 poles (97.1501, 17.9498) (96.6487, 17.9498) (96.1769, 18.7402) (96.1769, 19.5355) knots 0 0 0 1 2 2 2
  spline S117 degree 2 poles (96.7005, 20.4642) (96.6413, 20.3136) (96.5919, 19.8492) (96.5919, 19.5355) knots 0 0 0 1 2 2 2
  spline S118 degree 2 poles (96.5919, 19.5355) (96.5919, 19.2218) (96.6413, 18.7599) (96.703, 18.6043) knots 0 0 0 1 2 2 2
  spline S119 degree 2 poles (96.703, 18.6043) (96.7648, 18.4487) (96.9797, 18.2882) (97.1501, 18.2882) knots 0 0 0 1 2 2 2
  spline S120 degree 2 poles (97.1501, 18.2882) (97.3205, 18.2882) (97.5403, 18.4487) (97.6046, 18.6093) knots 0 0 0 1 2 2 2
  spline S121 degree 2 poles (97.6046, 18.6093) (97.6663, 18.7649) (97.7108, 19.2391) (97.7108, 19.538) knots 0 0 0 1 2 2 2
  spline S122 degree 2 poles (97.7108, 19.538) (97.7108, 19.8591) (97.6713, 20.2889) (97.607, 20.4568) knots 0 0 0 1 2 2 2
  spline S123 degree 2 poles (97.607, 20.4568) (97.5478, 20.6149) (97.3279, 20.7853) (97.1501, 20.7853) knots 0 0 0 1 2 2 2
  spline S124 degree 2 poles (97.1501, 20.7853) (96.9821, 20.7853) (96.7623, 20.6248) (96.7005, 20.4642) knots 0 0 0 1 2 2 2
  spline S125 degree 2 poles (94.8653, 21.1287) (95.0926, 21.1287) (95.4655, 20.9928) (95.5964, 20.8669) knots 0 0 0 1 2 2 2
  spline S126 degree 2 poles (95.5964, 20.8669) (95.7249, 20.7433) (95.8583, 20.4074) (95.8583, 20.2172) knots 0 0 0 1 2 2 2
  spline S127 degree 2 poles (95.8583, 20.2172) (95.8583, 19.9702) (95.594, 19.5553) (95.342, 19.4318) knots 0 0 0 1 2 2 2
  line L190 (95.342, 19.4318) -> (95.342, 19.4194)
  spline S128 degree 2 poles (95.342, 19.4194) (95.5668, 19.2885) (95.7842, 18.9773) (95.7842, 18.7451) knots 0 0 0 1 2 2 2
  spline S129 degree 2 poles (95.7842, 18.7451) (95.7842, 18.4018) (95.2655, 17.9424) (94.8653, 17.9424) knots 0 0 0 1 2 2 2
  spline S130 degree 2 poles (94.8653, 17.9424) (94.4504, 17.9424) (93.9489, 18.3771) (93.9489, 18.7179) knots 0 0 0 1 2 2 2
  spline S131 degree 2 poles (93.9489, 18.7179) (93.9489, 18.9229) (94.1885, 19.3231) (94.4133, 19.4367) knots 0 0 0 1 2 2 2
  line L191 (94.4133, 19.4367) -> (94.4133, 19.4491)
  spline S132 degree 2 poles (94.4133, 19.4491) (94.1465, 19.5726) (93.8724, 19.9282) (93.8724, 20.2098) knots 0 0 0 1 2 2 2
  spline S133 degree 2 poles (93.8724, 20.2098) (93.8724, 20.6001) (94.4405, 21.1287) (94.8653, 21.1287) knots 0 0 0 1 2 2 2
  spline S134 degree 2 poles (94.2923, 20.2493) (94.2923, 20.0616) (94.4405, 19.8393) (94.6504, 19.7257) knots 0 0 0 1 2 2 2
  spline S135 degree 2 poles (94.6504, 19.7257) (94.7196, 19.6862) (94.9518, 19.5948) (95.0975, 19.5355) knots 0 0 0 1 2 2 2
  spline S136 degree 2 poles (95.0975, 19.5355) (95.2655, 19.6467) (95.4458, 19.9776) (95.4458, 20.1876) knots 0 0 0 1 2 2 2
  spline S137 degree 2 poles (95.4458, 20.1876) (95.4458, 20.4642) (95.1123, 20.8249) (94.8604, 20.8249) knots 0 0 0 1 2 2 2
  spline S138 degree 2 poles (94.8604, 20.8249) (94.6035, 20.8249) (94.2923, 20.5161) (94.2923, 20.2493) knots 0 0 0 1 2 2 2
  spline S139 degree 2 poles (94.3491, 18.7229) (94.3491, 18.5179) (94.6233, 18.2437) (94.8678, 18.2437) knots 0 0 0 1 2 2 2
  spline S140 degree 2 poles (94.8678, 18.2437) (95.0901, 18.2437) (95.3741, 18.4882) (95.3741, 18.6982) knots 0 0 0 1 2 2 2
  spline S141 degree 2 poles (95.3741, 18.6982) (95.3741, 18.8488) (95.2284, 19.0588) (95.0827, 19.1428) knots 0 0 0 1 2 2 2
  spline S142 degree 2 poles (95.0827, 19.1428) (95.0209, 19.1774) (94.7591, 19.2984) (94.6529, 19.333) knots 0 0 0 1 2 2 2
  spline S143 degree 2 poles (94.6529, 19.333) (94.4751, 19.1971) (94.3491, 18.9081) (94.3491, 18.7229) knots 0 0 0 1 2 2 2
  line L192 (92.2323, 17.8757) -> (93.4253, 21.7215)
  line L193 (93.4253, 21.7215) -> (93.7711, 21.7215)
  line L194 (93.7711, 21.7215) -> (92.583, 17.8757)
  line L195 (92.583, 17.8757) -> (92.2323, 17.8757)
  line L196 (90.1698, 21.0595) -> (91.6568, 21.0595)
  line L197 (91.6568, 21.0595) -> (91.6568, 20.7483)
  line L198 (91.6568, 20.7483) -> (91.1035, 20.7483)
  line L199 (91.1035, 20.7483) -> (91.1035, 18.7056)
  line L200 (91.1035, 18.7056) -> (91.6568, 18.7056)
  line L201 (91.6568, 18.7056) -> (91.6568, 18.4265)
  spline S144 degree 2 poles (91.6568, 18.4265) (91.3431, 18.4265) (91.0467, 18.2486) (91.0269, 18.0016) knots 0 0 0 1 2 2 2
  line L202 (91.0269, 18.0016) -> (90.7108, 18.0016)
  line L203 (90.7108, 18.0016) -> (90.7108, 20.7483)
  line L204 (90.7108, 20.7483) -> (90.1698, 20.7483)
  line L205 (90.1698, 20.7483) -> (90.1698, 21.0595)
  spline S145 degree 2 poles (88.6878, 21.1287) (88.915, 21.1287) (89.288, 20.9928) (89.4189, 20.8669) knots 0 0 0 1 2 2 2
  spline S146 degree 2 poles (89.4189, 20.8669) (89.5474, 20.7433) (89.6808, 20.4074) (89.6808, 20.2172) knots 0 0 0 1 2 2 2
  spline S147 degree 2 poles (89.6808, 20.2172) (89.6808, 19.9702) (89.4165, 19.5553) (89.1645, 19.4318) knots 0 0 0 1 2 2 2
  line L206 (89.1645, 19.4318) -> (89.1645, 19.4194)
  spline S148 degree 2 poles (89.1645, 19.4194) (89.3893, 19.2885) (89.6067, 18.9773) (89.6067, 18.7451) knots 0 0 0 1 2 2 2
  spline S149 degree 2 poles (89.6067, 18.7451) (89.6067, 18.4018) (89.088, 17.9424) (88.6878, 17.9424) knots 0 0 0 1 2 2 2
  spline S150 degree 2 poles (88.6878, 17.9424) (88.2728, 17.9424) (87.7714, 18.3771) (87.7714, 18.7179) knots 0 0 0 1 2 2 2
  spline S151 degree 2 poles (87.7714, 18.7179) (87.7714, 18.9229) (88.011, 19.3231) (88.2358, 19.4367) knots 0 0 0 1 2 2 2
  line L207 (88.2358, 19.4367) -> (88.2358, 19.4491)
  spline S152 degree 2 poles (88.2358, 19.4491) (87.969, 19.5726) (87.6949, 19.9282) (87.6949, 20.2098) knots 0 0 0 1 2 2 2
  spline S153 degree 2 poles (87.6949, 20.2098) (87.6949, 20.6001) (88.263, 21.1287) (88.6878, 21.1287) knots 0 0 0 1 2 2 2
  spline S154 degree 2 poles (88.1148, 20.2493) (88.1148, 20.0616) (88.263, 19.8393) (88.4729, 19.7257) knots 0 0 0 1 2 2 2
  spline S155 degree 2 poles (88.4729, 19.7257) (88.5421, 19.6862) (88.7743, 19.5948) (88.92, 19.5355) knots 0 0 0 1 2 2 2
  spline S156 degree 2 poles (88.92, 19.5355) (89.088, 19.6467) (89.2683, 19.9776) (89.2683, 20.1876) knots 0 0 0 1 2 2 2
  spline S157 degree 2 poles (89.2683, 20.1876) (89.2683, 20.4642) (88.9348, 20.8249) (88.6829, 20.8249) knots 0 0 0 1 2 2 2
  spline S158 degree 2 poles (88.6829, 20.8249) (88.426, 20.8249) (88.1148, 20.5161) (88.1148, 20.2493) knots 0 0 0 1 2 2 2
  spline S159 degree 2 poles (88.1716, 18.7229) (88.1716, 18.5179) (88.4457, 18.2437) (88.6903, 18.2437) knots 0 0 0 1 2 2 2
  spline S160 degree 2 poles (88.6903, 18.2437) (88.9126, 18.2437) (89.1966, 18.4882) (89.1966, 18.6982) knots 0 0 0 1 2 2 2
  spline S161 degree 2 poles (89.1966, 18.6982) (89.1966, 18.8488) (89.0509, 19.0588) (88.9052, 19.1428) knots 0 0 0 1 2 2 2
  spline S162 degree 2 poles (88.9052, 19.1428) (88.8434, 19.1774) (88.5816, 19.2984) (88.4754, 19.333) knots 0 0 0 1 2 2 2
  spline S163 degree 2 poles (88.4754, 19.333) (88.2975, 19.1971) (88.1716, 18.9081) (88.1716, 18.7229) knots 0 0 0 1 2 2 2
  line L208 (86.0548, 17.8757) -> (87.2478, 21.7215)
  line L209 (87.2478, 21.7215) -> (87.5936, 21.7215)
  line L210 (87.5936, 21.7215) -> (86.4055, 17.8757)
  line L211 (86.4055, 17.8757) -> (86.0548, 17.8757)
  line L212 (83.8392, 21.0595) -> (85.7188, 21.0595)
  line L213 (85.7188, 21.0595) -> (85.7188, 20.6273)
  spline S164 degree 2 poles (85.7188, 20.6273) (85.5163, 20.4371) (85.1557, 20.0839) (84.9828, 19.8937) knots 0 0 0 1 2 2 2
  spline S165 degree 2 poles (84.9828, 19.8937) (84.6345, 19.5108) (84.3801, 19.0514) (84.3801, 18.8069) knots 0 0 0 1 2 2 2
  spline S166 degree 2 poles (84.3801, 18.8069) (84.3801, 18.6784) (84.4591, 18.4858) (84.5308, 18.424) knots 0 0 0 1 2 2 2
  spline S167 degree 2 poles (84.5308, 18.424) (84.6024, 18.3623) (84.7901, 18.3005) (84.9037, 18.3005) knots 0 0 0 1 2 2 2
  spline S168 degree 2 poles (84.9037, 18.3005) (85.0124, 18.3005) (85.2347, 18.3548) (85.336, 18.3968) knots 0 0 0 1 2 2 2
  spline S169 degree 2 poles (85.336, 18.3968) (85.4224, 18.4314) (85.583, 18.5302) (85.6324, 18.5648) knots 0 0 0 1 2 2 2
  line L214 (85.6324, 18.5648) -> (85.6546, 18.5648)
  line L215 (85.6546, 18.5648) -> (85.6546, 18.1301)
  spline S170 degree 2 poles (85.6546, 18.1301) (85.5287, 18.0683) (85.0766, 17.9473) (84.8741, 17.9473) knots 0 0 0 1 2 2 2
  spline S171 degree 2 poles (84.8741, 17.9473) (84.4468, 17.9473) (83.9651, 18.3993) (83.9651, 18.7846) knots 0 0 0 1 2 2 2
  spline S172 degree 2 poles (83.9651, 18.7846) (83.9651, 18.9649) (84.0491, 19.2663) (84.1232, 19.3947) knots 0 0 0 1 2 2 2
  spline S173 degree 2 poles (84.1232, 19.3947) (84.1973, 19.5281) (84.4122, 19.7899) (84.5308, 19.9159) knots 0 0 0 1 2 2 2
  spline S174 degree 2 poles (84.5308, 19.9159) (84.7234, 20.1258) (85.1952, 20.5754) (85.336, 20.7063) knots 0 0 0 1 2 2 2
  line L216 (85.336, 20.7063) -> (83.8392, 20.7063)
  line L217 (83.8392, 20.7063) -> (83.8392, 21.0595)
  spline S175 degree 2 poles (81.584, 20.0913) (81.584, 20.3111) (81.7248, 20.6865) (81.8533, 20.8249) knots 0 0 0 1 2 2 2
  spline S176 degree 2 poles (81.8533, 20.8249) (81.9817, 20.9632) (82.3646, 21.1237) (82.6017, 21.1237) knots 0 0 0 1 2 2 2
  spline S177 degree 2 poles (82.6017, 21.1237) (82.819, 21.1237) (83.2439, 21.0274) (83.3995, 20.9508) knots 0 0 0 1 2 2 2
  line L218 (83.3995, 20.9508) -> (83.3995, 20.5186)
  line L219 (83.3995, 20.5186) -> (83.3699, 20.5186)
  spline S178 degree 2 poles (83.3699, 20.5186) (83.3229, 20.5532) (83.1476, 20.6421) (83.0414, 20.6816) knots 0 0 0 1 2 2 2
  spline S179 degree 2 poles (83.0414, 20.6816) (82.9203, 20.7236) (82.7202, 20.7705) (82.5943, 20.7705) knots 0 0 0 1 2 2 2
  spline S180 degree 2 poles (82.5943, 20.7705) (82.4708, 20.7705) (82.2386, 20.6816) (82.1546, 20.5853) knots 0 0 0 1 2 2 2
  spline S181 degree 2 poles (82.1546, 20.5853) (82.078, 20.4939) (81.999, 20.2518) (81.999, 20.0888) knots 0 0 0 1 2 2 2
  spline S182 degree 2 poles (81.999, 20.0888) (81.999, 19.9258) (82.0879, 19.7183) (82.1719, 19.6491) knots 0 0 0 1 2 2 2
  spline S183 degree 2 poles (82.1719, 19.6491) (82.2584, 19.5726) (82.5152, 19.5083) (82.6708, 19.5083) knots 0 0 0 1 2 2 2
  spline S184 degree 2 poles (82.6708, 19.5083) (82.8388, 19.5083) (83.1723, 19.5602) (83.2735, 19.5824) knots 0 0 0 1 2 2 2
  line L220 (83.2735, 19.5824) -> (83.2735, 18.0115)
  line L221 (83.2735, 18.0115) -> (81.6013, 18.0115)
  line L222 (81.6013, 18.0115) -> (81.6013, 18.3697)
  line L223 (81.6013, 18.3697) -> (82.8808, 18.3697)
  line L224 (82.8808, 18.3697) -> (82.8808, 19.1823)
  spline S185 degree 2 poles (82.8808, 19.1823) (82.8067, 19.1724) (82.6634, 19.165) (82.6042, 19.165) knots 0 0 0 1 2 2 2
  spline S186 degree 2 poles (82.6042, 19.165) (82.3695, 19.165) (82.0459, 19.2416) (81.8977, 19.3552) knots 0 0 0 1 2 2 2
  spline S187 degree 2 poles (81.8977, 19.3552) (81.7471, 19.4688) (81.584, 19.8146) (81.584, 20.0913) knots 0 0 0 1 2 2 2
  point P0 (50.375, 0)
  dimension "d0" = 115
  dimension "d1" = 115
  constraints: 2 other
extrude "Extrusion5" cut sketch "Sketch8" against normal blind 2
body "Solid1"
